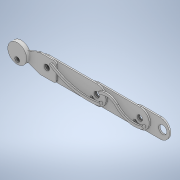
# Autodesk Inventor part: mozgasvizsgalat
Saved by Autodesk Inventor 2020 (Build 240168000, 168)
## iProperties
Created: 2019-08-09
Part Number: mozgasvizsgalat
Material: Generic
Document SubType Name: Modeling
Designer: Horváth Patrik
Density: 1 g/cm^3
Appearance: Default
Author: Horváth Patrik
Autodesk Inventor part; units mm, degrees
ref_plane "YZ Plane" through (0, 0, 0) normal (1, 0, 0) x (0, 1, 0)
ref_plane "XZ Plane" through (0, 0, 0) normal (0, 1, 0) x (-1, 0, 0)
ref_plane "XY Plane" through (0, 0, 0) normal (0, 0, 1) x (1, 0, 0)
sketch "Sketch1" plane through (0, 0, 0) normal (0, 0, 1) x (1, 0, 0)
  line L0 (-5, -7) -> (5, -7)
  line L1 (7, -5) -> (7, 5)
  line L2 (5, 7) -> (-5, 7)
  line L3 (-7, 5) -> (-7, -5)
  line L4 (-7, -7) -> (7, 7) construction
  line L5 (7, -7) -> (-7, 7) construction
  arc A0 (7, 5) -> (5, 7) centre (5, 5) ccw
  arc A1 (5, -7) -> (7, -5) centre (5, -5) ccw
  arc A2 (-7, -5) -> (-5, -7) centre (-5, -5) ccw
  arc A3 (-5, 7) -> (-7, 5) centre (-5, 5) ccw
  circle A4 centre (4, 4) radius 1
  circle A5 centre (0, 0) radius 2
  point P0 (0, 0)
  dimension "d0" = 14
  dimension "d1" = 2
  dimension "d2" = 2
  dimension "d3" = 3
  dimension "d6" = 4
  constraints: 12 end point, 9 point on line, 8 point on circle, 8 tangent, 6 centre point, 3 equal radius, 3 midpoint, 2 coincident, 2 parallel, 2 perpendicular, 1 horizontal
  measures "d0" distance of L4.end L5.end
  measures "d1" radius of A0
  measures "d2" diameter of A4
  measures "d3" distance from line of L1 A4.centre
  measures "d6" diameter of A5
extrude "Extrusion1" add sketch "Sketch1" along normal blind 1
sketch "Sketch2" plane through (0, 0, 0) normal (0, 0, -1) x (-1, 0, 0)
  line L0 (0, 0) -> (-36, 0) construction
  line L1 (0, -7) -> (-36, -7)
  line L2 (-36, 7) -> (0, 7)
  arc A0 (0, -7) -> (0, 7) centre (0, 0) ccw
  arc A1 (-36, 7) -> (-36, -7) centre (-36, 0) ccw
  line L3 (-5, 7) -> (5, 7) projected
  circle A2 centre (-36, 0) radius 2
  circle A3 centre (0, 0) radius 2 projected
  arc A4 (-39.5355, -3.5355) -> (-32.4645, -3.5355) centre (-36, 0) ccw construction
  arc A5 (-40.2426, -4.2426) -> (-31.7574, -4.2426) centre (-36, 0) ccw
  arc A6 (-38.8284, -2.8284) -> (-33.1716, -2.8284) centre (-36, 0) ccw
  arc A7 (-38.8284, -2.8284) -> (-40.2426, -4.2426) centre (-39.5355, -3.5355) ccw
  arc A8 (-31.7574, -4.2426) -> (-33.1716, -2.8284) centre (-32.4645, -3.5355) ccw
  line L4 (-36, 0) -> (-39.5355, -3.5355) construction
  line L5 (-32.4645, -3.5355) -> (-36, 0) construction
  line L6 (-36, 0) -> (-36, -7) construction
  circle A9 centre (-39, 3) radius 1
  point P0 (-18, 0)
  dimension "d7" = 50
  dimension "d8" = 90
  dimension "d9" = 2
  dimension "d10" = 5
  dimension "d11" = 2
  dimension "d12" = 3
  dimension "d13" = 3
  constraints: 14 end point, 14 point on circle, 9 centre point, 8 tangent, 2 coincident, 1 collinear, 1 equal radius, 1 horizontal, 1 midpoint, 1 parallel, 1 perpendicular, 1 other
  measures "d8" angle of L5 L4
  measures "d9" radial gap between concentric circles of A6 A5
  measures "d10" radius of A4
  measures "d11" diameter of A9
  measures "d12" horizontal distance of L0.end A9.centre
  measures "d13" horizontal distance of A9.centre L0.end
extrude "Extrusion2" add sketch "Sketch2" along normal blind 1 separate body
sketch "Sketch3" plane through (0, 0, -1) normal (0, 0, -1) x (-1, 0, 0)
  circle A0 centre (-36, 0) radius 2 projected
  line L0 (-36, 0) -> (-67, 0) construction
  line L1 (-36, 7) -> (-67, 7)
  line L2 (-67, -7) -> (-36, -7)
  arc A1 (-36, -7) -> (-36, 7) centre (-36, 0) ccw
  arc A2 (-67, 7) -> (-67, -7) centre (-67, 0) ccw
  line L3 (0, 7) -> (-36, 7) projected
  circle A3 centre (-67, 0) radius 2
  circle A4 centre (-36, 0) radius 2 projected
  circle A5 centre (-36, 0) radius 2
  arc A6 (-38.8284, -2.8284) -> (-40.2426, -4.2426) centre (-39.5355, -3.5355) ccw projected
  circle A7 centre (-39.5355, -3.5355) radius 1
  arc A8 (-70.5355, -3.5355) -> (-63.4645, -3.5355) centre (-67, 0) ccw construction
  arc A9 (-71.2426, -4.2426) -> (-62.7574, -4.2426) centre (-67, 0) ccw
  arc A10 (-69.8284, -2.8284) -> (-64.1716, -2.8284) centre (-67, 0) ccw
  arc A11 (-69.8284, -2.8284) -> (-71.2426, -4.2426) centre (-70.5355, -3.5355) ccw
  arc A12 (-62.7574, -4.2426) -> (-64.1716, -2.8284) centre (-63.4645, -3.5355) ccw
  line L4 (-67, 0) -> (-70.5355, -3.5355) construction
  line L5 (-67, 0) -> (-63.4645, -3.5355) construction
  line L6 (-67, 0) -> (-67, -7) construction
  point P0 (0, 0)
  point P1 (-51.5, 0)
  point P2 (-40.2426, -4.2426)
  point P3 (-38.8284, -2.8284)
  dimension "d17" = 31
  dimension "d18" = 2
  dimension "d19" = 90
  dimension "d20" = 5
  constraints: 14 end point, 14 point on circle, 10 centre point, 8 tangent, 4 coincident, 3 equal radius, 1 collinear, 1 midpoint, 1 parallel, 1 perpendicular, 1 vertical, 1 other
  measures "d17" distance of L0.start L0.end
  measures "d18" radial gap between concentric circles of A10 A9
  measures "d19" angle of L5 L4
  measures "d20" radius of A8
extrude "Extrusion3" add sketch "Sketch3" along normal blind 1 separate body
sketch "Sketch4" plane through (0, 0, -2) normal (0, 0, -1) x (-1, 0, 0)
  line L0 (-67, 0) -> (-81, 0) construction
  line L1 (-67, 7) -> (-81, 7)
  line L2 (-81, -7) -> (-67, -7)
  arc A0 (-67, -7) -> (-67, 7) centre (-67, 0) ccw
  arc A1 (-81, 7) -> (-81, -7) centre (-81, 0) ccw
  circle A2 centre (-67, 0) radius 2 projected
  arc A3 (-69.8284, -2.8284) -> (-71.2426, -4.2426) centre (-70.5355, -3.5355) ccw projected
  circle A4 centre (-70.5355, -3.5355) radius 1
  circle A5 centre (-67, 0) radius 2
  line L3 (-36, 7) -> (-67, 7) projected
  point P0 (0, 0)
  point P1 (-74, 0)
  point P2 (-71.2426, -4.2426)
  point P3 (-69.8284, -2.8284)
  dimension "d23" = 14
  constraints: 8 end point, 4 centre point, 4 point on circle, 4 tangent, 3 coincident, 2 concentric, 1 collinear, 1 midpoint, 1 parallel
  measures "d23" distance of L0.end L0.start
extrude "Extrusion4" add sketch "Sketch4" along normal blind 1 separate body
sketch "Sketch5" plane through (0, 0, 1) normal (0, 0, 1) x (1, 0, 0)
  circle A0 centre (4, 4) radius 1 projected
  circle A1 centre (39.5355, -3.5355) radius 1 projected
  arc A2 (4, 4) -> (39.5355, -3.5355) centre (31.4314, 45.8033) ccw construction
  arc A3 (3.4514, 3.1639) -> (39.6976, -4.5223) centre (31.4314, 45.8033) ccw
  arc A4 (4.5486, 4.8361) -> (39.3735, -2.5488) centre (31.4314, 45.8033) ccw
  arc A5 (4.5486, 4.8361) -> (3.4514, 3.1639) centre (4, 4) ccw
  arc A6 (39.6976, -4.5223) -> (39.3735, -2.5488) centre (39.5355, -3.5355) ccw
  point P0 (0, 0)
  point P1 (39.3735, -2.5488)
  point P2 (4.5486, 4.8361)
  point P3 (3.4514, 3.1639)
  dimension "d26" = 50
  constraints: 10 point on circle, 5 centre point, 4 tangent, 1 concentric
  measures "d26" radius of A2
extrude "Extrusion5" add sketch "Sketch5" along normal blind 1 separate body
sketch "Sketch6" plane through (0, 0, 1) normal (0, 0, -1) x (-1, 0, 0)
  circle A0 centre (-39.5355, -3.5355) radius 1 projected
  point P0 (0, 0)
extrude "Extrusion6" add sketch "Sketch6" along normal blind 3 bodies 5
sketch "Sketch7" plane through (0, 0, 0) normal (0, 0, 1) x (1, 0, 0)
  circle A0 centre (39, 3) radius 1 projected
  arc A1 (51.4767, 1.2322) -> (39, 3) centre (44.149, -5.5725) ccw construction
  arc A2 (52.2095, 1.9127) -> (38.4851, 3.8573) centre (44.149, -5.5725) ccw
  arc A3 (50.7439, 0.5518) -> (39.5149, 2.1427) centre (44.149, -5.5725) ccw
  arc A4 (50.7439, 0.5518) -> (52.2095, 1.9127) centre (51.4767, 1.2322) ccw construction
  arc A5 (38.4851, 3.8573) -> (39.5149, 2.1427) centre (39, 3) ccw
  arc A6 (71.2426, -4.2426) -> (69.8284, -2.8284) centre (70.5355, -3.5355) ccw projected
  arc A7 (51.4767, 1.2322) -> (70.5355, -3.5355) centre (64.6666, 13.4808) ccw construction
  arc A8 (50.7439, 0.5518) -> (70.8616, -4.4809) centre (64.6666, 13.4808) ccw
  arc A9 (52.2095, 1.9127) -> (70.2095, -2.5902) centre (64.6666, 13.4808) ccw
  arc A10 (52.2095, 1.9127) -> (50.7439, 0.5518) centre (51.4767, 1.2322) ccw construction
  arc A11 (70.8616, -4.4809) -> (70.2095, -2.5902) centre (70.5355, -3.5355) ccw
  point P0 (0, 0)
  point P1 (50.7439, 0.5518)
  point P2 (71.2426, -4.2426)
  point P3 (70.2095, -2.5902)
  point P4 (52.2095, 1.9127)
  point P5 (38.4851, 3.8573)
  point P6 (39.5149, 2.1427)
  dimension "d31" = 10
  dimension "d32" = 18
  dimension "d33" = 18
  constraints: 20 point on circle, 10 centre point, 9 tangent, 2 concentric
  measures "d31" radius of A1
  measures "d32" radius of A7
  measures "d33" horizontal distance of A9.end A2.start
extrude "Extrusion7" add sketch "Sketch7" along normal blind 1 separate body
sketch "Sketch8" plane through (0, 0, 0) normal (0, 0, -1) x (-1, 0, 0)
  circle A0 centre (-70.5355, -3.5355) radius 1 projected
  point P0 (0, 0)
extrude "Extrusion8" add sketch "Sketch8" along normal blind 3 bodies 6
sketch "Sketch9" plane through (0, 0, 0) normal (0, 0, 1) x (1, 0, 0)
  circle A0 centre (-20, 0) radius 7
  circle A1 centre (-20, -4) radius 1.75
  point P0 (0, 0)
  dimension "d38" = 14
  dimension "d39" = 20
  dimension "d40" = 3.5
  dimension "d41" = 4
  constraints: 2 centre point
  measures "d38" diameter of A0
  measures "d39" distance of point (0, 0) A0.centre
  measures "d40" diameter of A1
  measures "d41" distance of A0.centre A1.centre
extrude "Extrusion9" add sketch "Sketch9" along normal blind 3 separate body
sketch "Sketch10" plane through (0, 0, -1) normal (0, 0, -1) x (-1, 0, 0)
  circle A0 centre (0, -4) radius 1.75
  point P0 (0, 0)
  dimension "d44" = 3.5
  dimension "d45" = 4
  constraints: 1 centre point
  measures "d44" diameter of A0
  measures "d45" distance of point (0, 0) A0.centre
extrude "Extrusion10" cut sketch "Sketch10" against normal blind 3 bodies 2
sketch "Sketch11" plane through (0, 0, -1) normal (0, 0, -1) x (-1, 0, 0)
  circle A0 centre (20, -4) radius 1.75 projected
  arc A1 (0, -2.25) -> (0, -5.75) centre (0, -4) ccw
  arc A2 (20, -5.75) -> (20, -2.25) centre (20, -4) ccw
  circle A3 centre (0, -4) radius 1.75 projected
  line L0 (0, -2.25) -> (20, -2.25)
  circle A4 centre (0, -4) radius 1.75 projected
  line L1 (20, -5.75) -> (0, -5.75)
  point P0 (0, 0)
  point P1 (19.7404, -8.7306)
  point P2 (20, -5.75)
  point P3 (21.7363, -6.7813)
  point P4 (18.2637, -6.7813)
  point P5 (21.75, -4)
  point P6 (20, -5.75)
  constraints: 4 end point, 4 point on circle, 4 tangent, 2 centre point, 1 coincident, 1 horizontal, 1 parallel, 2 other
extrude "Extrusion11" add sketch "Sketch11" along normal blind 3 separate body
sketch "Sketch12" plane through (0, 0, 1) normal (0, 0, 1) x (1, 0, 0)
  circle A0 centre (-20, 0) radius 7 projected
  circle A1 centre (-20, 0) radius 1.3221
  line L0 (-20.4715, 1.2351) -> (-5.7132, 6.8685)
  arc A2 (-5, 7) -> (-7, 5) centre (-5, 5) ccw projected
  arc A3 (-7, -5) -> (-5, -7) centre (-5, -5) ccw projected
  line L1 (-5.7132, -6.8685) -> (-20.4715, -1.2351)
  line L2 (-7, 5) -> (-7, -5) projected
  point P0 (0, 0)
  point P1 (-14.0494, 3.6865)
  point P2 (-14.0494, -3.6865)
  point P3 (-18.2637, -6.7813)
  point P4 (-21.7363, -6.7813)
  constraints: 4 end point, 4 point on circle, 4 tangent, 1 centre point, 1 coincident
extrude "Extrusion12" add sketch "Sketch12" against normal blind 1 contours A0 L1 A1 L0 | A0 L0 A2 L2 A3 L1 | A1 picked at (-14.9324, 0.4289) bodies 1
sketch "Sketch13" plane through (0, 0, -2) normal (0, 0, 1) x (1, 0, 0)
  circle A0 centre (83, 0) radius 3
  point P0 (0, 0)
  constraints: 1 centre point
extrude "Extrusion13" cut sketch "Sketch13" against normal blind 10 bodies 4
body "Solid1"
body "Solid2"
body "Solid3"
body "Solid4"
body "Solid5"
body "Solid6"
body "Solid7"
body "Solid8"
